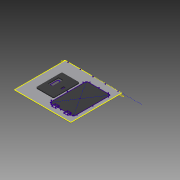
# Autodesk Inventor part: Right_side
Saved by Autodesk Inventor 2015 SP2 (Build 190223200, 223)
## iProperties
Created: 2016-11-11
Part Number: Right_side
Material: Generic
Document SubType Name: Modeling
Designer: Yann Cesbron
Density: 1 g/cm^3
Appearance: Default
Mass: 3388.49 g
Surface Area: 7563.24 cm^2
Volume: 3388.49 cm^3
Material: Perspex Black 9961 -10 mm
Author: Yann Cesbron
Autodesk Inventor part; units mm, degrees
ref_plane "YZ Plane" through (0, 0, 0) normal (1, 0, 0) x (0, 1, 0)
ref_plane "XZ Plane" through (0, 0, 0) normal (0, 1, 0) x (-1, 0, 0)
ref_plane "XY Plane" through (0, 0, 0) normal (0, 0, 1) x (1, 0, 0)
ref_plane "Work Plane1" through (5.6805, -10.8989, 0) normal (0, 0, 1) x (1, 0, 0)
sketch "Sketch1" plane through (5.6805, -10.8989, 0) normal (0, 0, 1) x (1, 0, 0)
  line L0 (-5.6805, 20.8989) -> (604.3195, 20.8989)
  line L1 (604.3195, 20.8989) -> (604.3195, -529.1011)
  line L2 (604.3195, -529.1011) -> (-5.6805, -529.1011)
  line L3 (-5.6805, -529.1011) -> (-5.6805, 20.8989)
  point P0 (-5.6805, 10.8989)
  dimension "d0" = 610
  dimension "d1" = 550
  dimension "d2" = 610
  dimension "d3" = 10
  constraints: 8 end point, 2 parallel, 1 horizontal, 1 perpendicular
  measures "d0" distance of L1.end L2.end
  measures "d1" distance of L0.end L1.end
  measures "d2" distance from line of point (-5.681, 10.899) L1
  measures "d3" distance from line of point (-5.681, 10.899) L0
extrude "Extrusion1" add sketch "Sketch1" along normal blind 10
sketch "Cut_out_right" plane through (5.6805, -10.8989, 10) normal (0, 0, 1) x (1, 0, 0)
  line L0 (604.3195, 20.8989) -> (-5.6805, 20.8989) projected
  line L1 (-5.6805, -529.1011) -> (604.3195, -529.1011) projected
  line L2 (274.3195, 20.8989) -> (824.3195, 20.8989) construction
  line L3 (-5.6805, 20.8989) -> (-5.6805, -529.1011) projected
  line L4 (264.3195, -134.1011) -> (124.3195, -134.1011)
  line L5 (114.3195, -144.1011) -> (114.3195, -374.1011)
  line L6 (124.3195, -384.1011) -> (264.3195, -384.1011)
  line L7 (274.3195, -374.1011) -> (274.3195, -144.1011)
  line L8 (274.3195, -134.1011) -> (114.3195, -384.1011) construction
  line L9 (114.3195, -134.1011) -> (274.3195, -384.1011) construction
  arc A0 (264.3195, -384.1011) -> (274.3195, -374.1011) centre (264.3195, -374.1011) ccw
  arc A1 (274.3195, -144.1011) -> (264.3195, -134.1011) centre (264.3195, -144.1011) ccw
  arc A2 (124.3195, -134.1011) -> (114.3195, -144.1011) centre (124.3195, -144.1011) ccw
  arc A3 (114.3195, -374.1011) -> (124.3195, -384.1011) centre (124.3195, -374.1011) ccw
  line L10 (314.3195, -459.1011) -> (554.3195, -459.1011)
  line L11 (564.3195, -449.1011) -> (564.3195, -69.1011)
  line L12 (554.3195, -59.1011) -> (314.3195, -59.1011)
  line L13 (304.3195, -69.1011) -> (304.3195, -449.1011)
  line L14 (304.3195, -459.1011) -> (564.3195, -59.1011) construction
  line L15 (564.3195, -459.1011) -> (304.3195, -59.1011) construction
  line L16 (604.3195, 20.8989) -> (604.3195, -529.1011) projected
  arc A4 (304.3195, -449.1011) -> (314.3195, -459.1011) centre (314.3195, -449.1011) ccw
  arc A5 (564.3195, -69.1011) -> (554.3195, -59.1011) centre (554.3195, -69.1011) ccw
  arc A6 (314.3195, -59.1011) -> (304.3195, -69.1011) centre (314.3195, -69.1011) ccw
  arc A7 (554.3195, -459.1011) -> (564.3195, -449.1011) centre (554.3195, -449.1011) ccw
  circle A8 centre (281.8195, -149.1011) radius 1.65
  circle A9 centre (259.3195, -126.6011) radius 1.65
  circle A10 centre (281.8195, -369.1011) radius 1.65
  circle A11 centre (281.8195, -259.1011) radius 1.65
  circle A12 centre (194.3195, -126.6011) radius 1.65
  circle A13 centre (129.3195, -126.6011) radius 1.65
  circle A14 centre (106.8195, -149.1011) radius 1.65
  circle A15 centre (106.8195, -259.1011) radius 1.65
  circle A16 centre (106.8195, -369.1011) radius 1.65
  circle A17 centre (129.3195, -391.6011) radius 1.65
  circle A18 centre (259.3195, -391.6011) radius 1.65
  circle A19 centre (194.3195, -391.6011) radius 1.65
  circle A20 centre (352.9195, -471.8011) radius 1.65
  circle A21 centre (384.7195, -471.8011) radius 1.65
  circle A22 centre (515.7195, -471.8011) radius 1.65
  circle A23 centre (483.9195, -471.8011) radius 1.65
  circle A24 centre (534.3195, -466.6011) radius 1.65
  circle A25 centre (434.3195, -466.6011) radius 1.65
  circle A26 centre (334.3195, -466.6011) radius 1.65
  circle A27 centre (296.8195, -429.1011) radius 1.65
  circle A28 centre (296.8195, -259.1011) radius 1.65
  circle A29 centre (296.8195, -89.1011) radius 1.65
  circle A30 centre (334.3195, -51.6011) radius 1.65
  circle A31 centre (434.3195, -51.6011) radius 1.65
  circle A32 centre (534.3195, -51.6011) radius 1.65
  circle A33 centre (571.8195, -89.1011) radius 1.65
  circle A34 centre (571.8195, -259.1011) radius 1.65
  circle A35 centre (571.8195, -429.1011) radius 1.65
  circle A36 centre (569.3195, 15.8989) radius 2.25
  circle A37 centre (434.3195, 15.8989) radius 2.25
  circle A38 centre (299.3195, 15.8989) radius 2.25
  circle A39 centre (164.3195, 15.8989) radius 2.25
  circle A40 centre (29.3195, 15.8989) radius 2.25
  point P0 (-5.6805, 10.8989)
  point P1 (194.3195, -259.1011)
  point P2 (434.3195, -259.1011)
  dimension "d29" = 160
  dimension "d30" = 250
  dimension "d31" = 280
  dimension "d32" = 155
  dimension "d33" = 10
  dimension "d34" = 260
  dimension "d35" = 400
  dimension "d36" = 40
  dimension "d37" = 80
  dimension "d38" = 10
  dimension "d39" = 310
  dimension "d43" = 30
  dimension "d44" = 3.3
  dimension "d45" = 7.5
  dimension "d46" = 15
  dimension "d47" = 3.3
  dimension "d48" = 7.5
  dimension "d49" = 15
  dimension "d64" = 3.3
  dimension "d65" = 3.3
  dimension "d66" = 3.3
  dimension "d67" = 3.3
  dimension "d68" = 3.3
  dimension "d69" = 3.3
  dimension "d70" = 3.3
  dimension "d71" = 3.3
  dimension "d72" = 3.3
  dimension "d73" = 3.3
  dimension "d74" = 7.5
  dimension "d75" = 7.5
  dimension "d76" = 7.5
  dimension "d77" = 7.5
  dimension "d78" = 7.5
  dimension "d79" = 7.5
  dimension "d80" = 7.5
  dimension "d81" = 7.5
  dimension "d82" = 7.5
  dimension "d83" = 7.5
  dimension "d84" = 15
  dimension "d85" = 15
  dimension "d86" = 15
  dimension "d87" = 15
  dimension "d88" = 15
  dimension "d89" = 15
  dimension "d90" = 125
  dimension "d91" = 125
  dimension "d92" = 80
  dimension "d93" = 80
  dimension "d169" = 3.3
  dimension "d170" = 3.3
  dimension "d171" = 3.3
  dimension "d172" = 3.3
  dimension "d173" = 31.8
  dimension "d174" = 31.8
  dimension "d175" = 48.6
  dimension "d176" = 48.6
  dimension "d177" = 12.7
  dimension "d178" = 12.7
  dimension "d179" = 12.7
  dimension "d180" = 12.7
  dimension "d181" = 3.3
  dimension "d182" = 3.3
  dimension "d183" = 3.3
  dimension "d184" = 3.3
  constraints: 41 centre point, 26 end point, 17 point on line, 16 point on circle, 16 tangent, 6 equal radius, 4 midpoint, 4 parallel, 3 horizontal, 2 perpendicular
  measures "d29" distance of L9.end L8.end
  measures "d30" distance of L8.end L9.start
  measures "d31" distance between parallel lines of L3 L7
  measures "d32" distance between parallel lines of L0 L4
  measures "d33" radius of A0
  measures "d34" distance of L15.end L14.end
  measures "d35" distance of L14.end L15.start
  measures "d36" distance between parallel lines of L16 L11
  measures "d37" distance between parallel lines of L0 L12
  measures "d38" radius of A4
  measures "d39" distance between parallel lines of L3 L13
  measures "d43" distance between parallel lines of L7 L13
  measures "d44" diameter of A8
  measures "d45" distance from line of L7 A8.centre
  measures "d46" distance from line of A8.centre L4
  measures "d47" diameter of A9
  measures "d48" distance from line of L4 A9.centre
  measures "d49" distance from line of A9.centre L7
  measures "d64" diameter of A10
  measures "d65" diameter of A11
  measures "d66" diameter of A12
  measures "d67" diameter of A13
  measures "d68" diameter of A14
  measures "d69" diameter of A15
  measures "d70" diameter of A16
  measures "d71" diameter of A17
  measures "d72" diameter of A18
  measures "d73" diameter of A19
  measures "d74" distance from line of L4 A12.centre
  measures "d75" distance from line of L4 A13.centre
  measures "d76" distance from line of L7 A11.centre
  measures "d77" distance from line of L5 A14.centre
  measures "d78" distance from line of L5 A15.centre
  measures "d79" distance from line of L5 A16.centre
  measures "d80" distance from line of L6 A17.centre
  measures "d81" distance from line of L6 A19.centre
  measures "d82" distance from line of L7 A10.centre
  measures "d83" distance from line of L6 A18.centre
  measures "d84" distance from line of L7 A18.centre
  measures "d85" distance from line of L5 A17.centre
  measures "d86" distance from line of L5 A13.centre
  measures "d87" distance from line of L4 A14.centre
  measures "d88" distance from line of L6 A16.centre
  measures "d89" distance from line of L6 A10.centre
  measures "d90" distance from line of L4 A11.centre
  measures "d91" distance from line of L6 A15.centre
  measures "d92" distance from line of L5 A12.centre
  measures "d93" distance from line of L7 A19.centre
  measures "d169" diameter of A20
  measures "d170" diameter of A21
  measures "d171" diameter of A22
  measures "d172" diameter of A23
  measures "d173" distance of A23.centre A22.centre
  measures "d174" distance of A20.centre A21.centre
  measures "d175" distance from line of A20.centre L13
  measures "d176" distance from line of A22.centre L11
  measures "d177" distance from line of L10 A22.centre
  measures "d178" distance from line of L10 A23.centre
  measures "d179" distance from line of L10 A21.centre
  measures "d180" distance from line of L10 A20.centre
  measures "d181" diameter of A24
  measures "d182" diameter of A25
  measures "d183" diameter of A26
  measures "d184" diameter of A27
sketch "Panel_right_holes_right" plane through (0, -540, 0) normal (0, -1, 0) x (1, 0, 0)
  circle A0 centre (575, 5) radius 1.65
  circle A1 centre (440, 5) radius 1.65
  circle A2 centre (305, 5) radius 1.65
  circle A3 centre (170, 5) radius 1.65
  circle A4 centre (35, 5) radius 1.65
  line L0 (0, 0) -> (0, 10) projected
  line L1 (610, 0) -> (0, 0) projected
  line L2 (610, 0) -> (610, 10) projected
  dimension "d256" = 3.3
  dimension "d257" = 3.3
  dimension "d258" = 3.3
  dimension "d259" = 3.3
  dimension "d260" = 3.3
  dimension "d261" = 35
  dimension "d262" = 5
  dimension "d263" = 5
  dimension "d264" = 135
  dimension "d265" = 135
  dimension "d266" = 5
  dimension "d268" = 5
  dimension "d269" = 35
  dimension "d270" = 5
  dimension "d271" = 135
  constraints: 5 centre point
  measures "d256" diameter of A0
  measures "d257" diameter of A1
  measures "d258" diameter of A2
  measures "d259" diameter of A3
  measures "d260" diameter of A4
  measures "d261" distance from line of L0 A4.centre
  measures "d262" distance from line of L1 A4.centre
  measures "d263" distance from line of L1 A3.centre
  measures "d264" distance of A4.centre A3.centre
  measures "d265" distance of A2.centre A3.centre
  measures "d266" distance from line of L1 A2.centre
  measures "d268" distance from line of L1 A1.centre
  measures "d269" distance from line of L2 A0.centre
  measures "d270" distance from line of L1 A0.centre
  measures "d271" distance of A1.centre A0.centre
sketch "Panel_top_holes_right" plane through (610, -540, 0) normal (1, 0, 0) x (0, 0, -1)
  circle A0 centre (-5, 515) radius 1.65
  circle A1 centre (-5, 355) radius 1.65
  circle A2 centre (-5, 195) radius 1.65
  circle A3 centre (-5, 35) radius 1.65
  line L0 (-10, 0) -> (-10, 550) projected
  line L1 (0, 0) -> (-10, 0) projected
  line L2 (0, 550) -> (-10, 550) projected
  point P0 (0, 540)
  dimension "d272" = 3.3
  dimension "d273" = 3.3
  dimension "d274" = 3.3
  dimension "d275" = 3.3
  dimension "d276" = 5
  dimension "d277" = 35
  dimension "d278" = 5
  dimension "d279" = 160
  dimension "d280" = 5
  dimension "d281" = 5
  dimension "d282" = 35
  dimension "d283" = 160
  dimension "d284" = 160
  constraints: 4 centre point
  measures "d272" diameter of A0
  measures "d273" diameter of A1
  measures "d274" diameter of A2
  measures "d275" diameter of A3
  measures "d276" distance from line of L0 A3.centre
  measures "d277" distance from line of L1 A3.centre
  measures "d278" distance from line of L0 A2.centre
  measures "d279" distance of A3.centre A2.centre
  measures "d280" distance from line of L0 A0.centre
  measures "d281" distance from line of L0 A1.centre
  measures "d282" distance from line of A0.centre L2
  measures "d283" distance of A1.centre A0.centre
  measures "d284" distance of A2.centre A1.centre
extrude "Extrusion2" cut sketch "Cut_out_right" against normal blind 10 keep common part
extrude "Extrusion6" cut sketch "Panel_top_holes_right" against normal blind 15
extrude "Extrusion5" cut sketch "Panel_right_holes_right" against normal blind 15
sketch "Bracket_holes_right" plane through (5.6805, -10.8989, 10) normal (0, 0, 1) x (1, 0, 0)
  line L0 (-5.6805, 20.8989) -> (-5.6805, -529.1011) projected
  line L1 (-5.6805, -529.1011) -> (604.3195, -529.1011) projected
  line L2 (604.3195, 20.8989) -> (-5.6805, 20.8989) projected
  point P0 (-5.6805, 10.8989)
  point P1 (1.8195, -109.1011)
  point P2 (1.8195, -409.1011)
  dimension "d562" = 7.5
  dimension "d563" = 120
  dimension "d564" = 7.5
  dimension "d565" = 130
  measures "d562" distance from line of L0 point (1.819, -409.101)
  measures "d563" distance from line of L1 point (1.819, -409.101)
  measures "d564" distance from line of L0 point (1.819, -109.101)
  measures "d565" distance from line of L2 point (1.819, -109.101)
hole "Bracket_holes_right_1" at (7.5, -120, 10) at (7.5, -420, 10) direction (0, 0, -1) diameter 3.3 end through all
sketch "CRISP+X-motor" plane through (5.6805, -10.8989, 10) normal (0, 0, 1) x (1, 0, 0)
  circle A0 centre (250.3195, -259.1011) radius 8
  line L0 (138.3195, -204.1011) -> (168.4695, -204.1011)
  line L1 (168.4695, -204.1011) -> (168.4695, -289.2011)
  line L2 (168.4695, -289.2011) -> (138.3195, -289.2011)
  line L3 (138.3195, -289.2011) -> (138.3195, -204.1011)
  line L4 (604.3195, 20.8989) -> (-5.6805, 20.8989) projected
  line L5 (-5.6805, 20.8989) -> (-5.6805, -529.1011) projected
  line L6 (242.7195, -242.6011) -> (257.9195, -242.6011)
  line L7 (257.9195, -242.6011) -> (257.9195, -275.6011)
  line L8 (257.9195, -275.6011) -> (242.7195, -275.6011)
  line L9 (242.7195, -275.6011) -> (242.7195, -242.6011)
  line L10 (242.7195, -242.6011) -> (257.9195, -275.6011) construction
  line L11 (257.9195, -242.6011) -> (242.7195, -275.6011) construction
  point P0 (-5.6805, 10.8989)
  dimension "d19" = 16
  dimension "d20" = 30.15
  dimension "d21" = 85.1
  dimension "d22" = 280
  dimension "d23" = 256
  dimension "d24" = 225
  dimension "d25" = 144
  dimension "d41" = 33
  dimension "d42" = 15.2
  constraints: 20 end point, 4 parallel, 2 horizontal, 2 midpoint, 2 perpendicular, 1 centre point
  measures "d19" diameter of A0
  measures "d20" distance of L1.end L2.end
  measures "d21" distance of L0.end L1.end
  measures "d22" distance from line of L4 A0.centre
  measures "d23" distance from line of L5 A0.centre
  measures "d24" distance from line of L4 L0.start
  measures "d25" distance between parallel lines of L5 L3
  measures "d41" distance of L6.end L7.end
  measures "d42" distance between parallel lines of L9 L7
sketch "Hinges_right" plane through (5.6805, -10.8989, 10) normal (0, 0, 1) x (1, 0, 0)
  line L0 (524.3195, -481.1011) -> (475.3195, -481.1011)
  line L1 (475.3195, -481.1011) -> (475.3195, -437.1011)
  line L2 (475.3195, -437.1011) -> (524.3195, -437.1011)
  line L3 (524.3195, -437.1011) -> (524.3195, -481.1011)
  line L4 (344.3195, -481.1011) -> (393.3195, -481.1011)
  line L5 (393.3195, -481.1011) -> (393.3195, -437.1011)
  line L6 (393.3195, -437.1011) -> (344.3195, -437.1011)
  line L7 (344.3195, -437.1011) -> (344.3195, -481.1011)
  line L8 (-5.6805, -529.1011) -> (604.3195, -529.1011) projected
  line L9 (604.3195, -529.1011) -> (604.3195, 20.8989) projected
  circle A0 centre (515.7195, -446.4011) radius 2.25
  circle A1 centre (483.9195, -446.4011) radius 2.25
  circle A2 centre (515.7195, -471.8011) radius 2.25
  circle A3 centre (483.9195, -471.8011) radius 2.25
  circle A4 centre (352.9195, -471.8011) radius 2.25
  circle A5 centre (352.9195, -446.4011) radius 2.25
  circle A6 centre (384.7195, -446.4011) radius 2.25
  circle A7 centre (384.7195, -471.8011) radius 2.25
  point P0 (-5.6805, 10.8989)
  dimension "d130" = 49
  dimension "d131" = 44
  dimension "d132" = 49
  dimension "d133" = 44
  dimension "d143" = 80
  dimension "d144" = 260
  dimension "d145" = 4.5
  dimension "d146" = 4.5
  dimension "d147" = 4.5
  dimension "d148" = 4.5
  dimension "d149" = 4.5
  dimension "d150" = 4.5
  dimension "d151" = 4.5
  dimension "d152" = 4.5
  dimension "d153" = 9.3
  dimension "d154" = 9.3
  dimension "d155" = 8.6
  dimension "d156" = 8.6
  dimension "d157" = 8.6
  dimension "d158" = 8.6
  dimension "d159" = 9.3
  dimension "d160" = 9.3
  dimension "d161" = 8.6
  dimension "d162" = 8.6
  dimension "d163" = 8.6
  dimension "d164" = 8.6
  dimension "d165" = 9.3
  dimension "d166" = 9.3
  dimension "d167" = 9.3
  dimension "d168" = 9.3
  dimension "d239" = 48
  dimension "d240" = 48
  constraints: 16 end point, 8 centre point, 4 parallel, 2 horizontal, 2 perpendicular
  measures "d130" distance of L1.end L2.end
  measures "d131" distance of L0.end L1.end
  measures "d132" distance of L6.end L5.end
  measures "d133" distance of L5.end L4.end
  measures "d143" distance between parallel lines of L9 L3
  measures "d144" distance between parallel lines of L7 L9
  measures "d145" diameter of A0
  measures "d146" diameter of A1
  measures "d147" diameter of A2
  measures "d148" diameter of A3
  measures "d149" diameter of A4
  measures "d150" diameter of A5
  measures "d151" diameter of A6
  measures "d152" diameter of A7
  measures "d153" distance from line of L0 A2.centre
  measures "d154" distance from line of L0 A3.centre
  measures "d155" distance from line of L3 A2.centre
  measures "d156" distance from line of L3 A0.centre
  measures "d157" distance from line of L1 A1.centre
  measures "d158" distance from line of L1 A3.centre
  measures "d159" distance from line of L2 A0.centre
  measures "d160" distance from line of L2 A1.centre
  measures "d161" distance from line of L5 A6.centre
  measures "d162" distance from line of L5 A7.centre
  measures "d163" distance from line of L7 A5.centre
  measures "d164" distance from line of L7 A4.centre
  measures "d165" distance from line of L4 A4.centre
  measures "d166" distance from line of L6 A5.centre
  measures "d167" distance from line of L6 A6.centre
  measures "d168" distance from line of L4 A7.centre
  measures "d239" distance between parallel lines of L8 L0
  measures "d240" distance between parallel lines of L8 L4
sketch "Flange_right" plane through (5.6805, -10.8989, 10) normal (0, 0, 1) x (1, 0, 0)
  line L0 (279.3195, -119.1011) -> (109.3195, -119.1011)
  line L1 (99.3195, -129.1011) -> (99.3195, -389.1011)
  line L2 (109.3195, -399.1011) -> (279.3195, -399.1011)
  line L3 (289.3195, -389.1011) -> (289.3195, -129.1011)
  line L4 (289.3195, -119.1011) -> (99.3195, -399.1011) construction
  line L5 (99.3195, -119.1011) -> (289.3195, -399.1011) construction
  line L6 (604.3195, 20.8989) -> (-5.6805, 20.8989) projected
  line L7 (-5.6805, 20.8989) -> (-5.6805, -529.1011) projected
  line L8 (128.3195, -184.1011) -> (178.4695, -184.1011)
  line L9 (178.4695, -184.1011) -> (178.4695, -299.2011)
  line L10 (178.4695, -299.2011) -> (128.3195, -299.2011)
  line L11 (128.3195, -299.2011) -> (128.3195, -184.1011)
  line L12 (260.3195, -240.1011) -> (240.3195, -240.1011)
  line L13 (240.3195, -240.1011) -> (240.3195, -278.1011)
  line L14 (240.3195, -278.1011) -> (260.3195, -278.1011)
  line L15 (260.3195, -278.1011) -> (260.3195, -240.1011)
  line L16 (260.3195, -240.1011) -> (240.3195, -278.1011) construction
  line L17 (240.3195, -240.1011) -> (260.3195, -278.1011) construction
  circle A0 centre (194.3195, -126.6011) radius 2.25
  circle A1 centre (259.3195, -126.6011) radius 2.25
  circle A2 centre (281.8195, -149.1011) radius 2.25
  circle A3 centre (281.8195, -259.1011) radius 2.25
  circle A4 centre (281.8195, -369.1011) radius 2.25
  circle A5 centre (259.3195, -391.6011) radius 2.25
  circle A6 centre (194.3195, -391.6011) radius 2.25
  circle A7 centre (129.3195, -391.6011) radius 2.25
  circle A8 centre (106.8195, -369.1011) radius 2.25
  circle A9 centre (106.8195, -259.1011) radius 2.25
  circle A10 centre (106.8195, -149.1011) radius 2.25
  circle A11 centre (129.3195, -126.6011) radius 2.25
  arc A12 (289.3195, -129.1011) -> (279.3195, -119.1011) centre (279.3195, -129.1011) ccw
  arc A13 (279.3195, -399.1011) -> (289.3195, -389.1011) centre (279.3195, -389.1011) ccw
  arc A14 (109.3195, -119.1011) -> (99.3195, -129.1011) centre (109.3195, -129.1011) ccw
  arc A15 (99.3195, -389.1011) -> (109.3195, -399.1011) centre (109.3195, -389.1011) ccw
  point P0 (-5.6805, 10.8989)
  point P1 (194.3195, -259.1011)
  point P2 (250.3195, -259.1011)
  dimension "d51" = 190
  dimension "d52" = 280
  dimension "d53" = 280
  dimension "d54" = 200
  dimension "d55" = 50.15
  dimension "d56" = 65
  dimension "d57" = 29
  dimension "d58" = 115.1
  dimension "d59" = 20
  dimension "d60" = 38
  dimension "d62" = 39
  dimension "d63" = 140
  dimension "d94" = 4.5
  dimension "d95" = 4.5
  dimension "d96" = 4.5
  dimension "d97" = 4.5
  dimension "d98" = 4.5
  dimension "d99" = 4.5
  dimension "d100" = 4.5
  dimension "d101" = 4.5
  dimension "d102" = 4.5
  dimension "d103" = 4.5
  dimension "d104" = 4.5
  dimension "d105" = 4.5
  dimension "d106" = 7.5
  dimension "d107" = 30
  dimension "d108" = 7.5
  dimension "d109" = 140
  dimension "d110" = 7.5
  dimension "d111" = 30
  dimension "d112" = 7.5
  dimension "d113" = 7.5
  dimension "d114" = 7.5
  dimension "d115" = 7.5
  dimension "d116" = 7.5
  dimension "d117" = 30
  dimension "d118" = 30
  dimension "d119" = 30
  dimension "d120" = 30
  dimension "d121" = 7.5
  dimension "d122" = 7.5
  dimension "d123" = 7.5
  dimension "d124" = 7.5
  dimension "d125" = 30
  dimension "d126" = 30
  dimension "d127" = 140
  dimension "d128" = 95
  dimension "d129" = 95
  dimension "d217" = 10
  constraints: 32 end point, 16 centre point, 8 point on circle, 8 point on line, 8 tangent, 6 parallel, 4 midpoint, 3 equal radius, 3 horizontal, 3 perpendicular
  measures "d51" distance of L5.end L4.end
  measures "d52" distance of L4.end L5.start
  measures "d53" distance from line of L6 point (194.319, -259.101)
  measures "d54" distance from line of L7 point (194.319, -259.101)
  measures "d55" distance of L9.end L10.end
  measures "d56" distance between parallel lines of L0 L8
  measures "d57" distance between parallel lines of L1 L11
  measures "d58" distance between parallel lines of L10 L8
  measures "d59" distance of L14.end L13.end
  measures "d60" distance of L13.end L12.end
  measures "d62" distance from line of L3 point (250.319, -259.101)
  measures "d63" distance from line of L0 point (250.319, -259.101)
  measures "d94" diameter of A0
  measures "d95" diameter of A1
  measures "d96" diameter of A2
  measures "d97" diameter of A3
  measures "d98" diameter of A4
  measures "d99" diameter of A5
  measures "d100" diameter of A6
  measures "d101" diameter of A7
  measures "d102" diameter of A8
  measures "d103" diameter of A9
  measures "d104" diameter of A10
  measures "d105" diameter of A11
  measures "d106" distance from line of L3 A2.centre
  measures "d107" distance from line of L0 A2.centre
  measures "d108" distance from line of L3 A3.centre
  measures "d109" distance from line of L0 A3.centre
  measures "d110" distance from line of L3 A4.centre
  measures "d111" distance from line of L2 A4.centre
  measures "d112" distance from line of L2 A5.centre
  measures "d113" distance from line of L2 A6.centre
  measures "d114" distance from line of L0 A1.centre
  measures "d115" distance from line of L0 A0.centre
  measures "d116" distance from line of L0 A11.centre
  measures "d117" distance from line of L3 A1.centre
  measures "d118" distance from line of L1 A11.centre
  measures "d119" distance from line of L3 A5.centre
  measures "d120" distance from line of L1 A7.centre
  measures "d121" distance from line of L2 A7.centre
  measures "d122" distance from line of L1 A8.centre
  measures "d123" distance from line of L1 A10.centre
  measures "d124" distance from line of L1 A9.centre
  measures "d125" distance from line of A10.centre L0
  measures "d126" distance from line of L2 A8.centre
  measures "d127" distance from line of L2 A9.centre
  measures "d128" distance from line of L3 A6.centre
  measures "d129" distance from line of L1 A0.centre
  measures "d217" radius of A12
sketch "Door_right" plane through (5.6805, -10.8989, 10) normal (0, 0, 1) x (1, 0, 0)
  line L0 (554.3195, -457.1011) -> (314.3195, -457.1011)
  line L1 (306.3195, -449.1011) -> (306.3195, -69.1011)
  line L2 (314.3195, -61.1011) -> (554.3195, -61.1011)
  line L3 (562.3195, -69.1011) -> (562.3195, -449.1011)
  line L4 (562.3195, -457.1011) -> (306.3195, -61.1011) construction
  line L5 (306.3195, -457.1011) -> (562.3195, -61.1011) construction
  arc A0 (562.3195, -69.1011) -> (554.3195, -61.1011) centre (554.3195, -69.1011) ccw
  arc A1 (314.3195, -61.1011) -> (306.3195, -69.1011) centre (314.3195, -69.1011) ccw
  arc A2 (306.3195, -449.1011) -> (314.3195, -457.1011) centre (314.3195, -449.1011) ccw
  arc A3 (554.3195, -457.1011) -> (562.3195, -449.1011) centre (554.3195, -449.1011) ccw
  circle A4 centre (515.7195, -446.4011) radius 1.65
  circle A5 centre (483.9195, -446.4011) radius 1.65
  circle A6 centre (384.7195, -446.4011) radius 1.65
  circle A7 centre (352.9195, -446.4011) radius 1.65
  line L6 (-5.6805, 20.8989) -> (-5.6805, -529.1011) projected
  line L7 (604.3195, 20.8989) -> (-5.6805, 20.8989) projected
  point P0 (-5.6805, 10.8989)
  point P1 (434.3195, -259.1011)
  dimension "d218" = 256
  dimension "d219" = 396
  dimension "d220" = 8
  dimension "d221" = 8
  dimension "d222" = 8
  dimension "d223" = 8
  dimension "d224" = 3.3
  dimension "d225" = 3.3
  dimension "d226" = 3.3
  dimension "d227" = 3.3
  dimension "d228" = 10.7
  dimension "d229" = 10.7
  dimension "d230" = 31.8
  dimension "d231" = 10.7
  dimension "d232" = 10.7
  dimension "d233" = 31.8
  dimension "d234" = 46.6
  dimension "d235" = 46.6
  dimension "d236" = 440
  dimension "d237" = 280
  constraints: 12 end point, 8 centre point, 8 point on circle, 8 point on line, 8 tangent, 2 midpoint, 2 parallel, 1 horizontal, 1 perpendicular
  measures "d218" distance of L4.end L5.end
  measures "d219" distance of L5.start L4.end
  measures "d220" radius of A0
  measures "d221" radius of A1
  measures "d222" radius of A2
  measures "d223" radius of A3
  measures "d224" diameter of A4
  measures "d225" diameter of A5
  measures "d226" diameter of A6
  measures "d227" diameter of A7
  measures "d228" distance from line of L0 A4.centre
  measures "d229" distance from line of L0 A5.centre
  measures "d230" distance of A4.centre A5.centre
  measures "d231" distance from line of L0 A6.centre
  measures "d232" distance from line of L0 A7.centre
  measures "d233" distance of A7.centre A6.centre
  measures "d234" distance from line of L1 A7.centre
  measures "d235" distance from line of L3 A4.centre
  measures "d236" distance from line of L6 point (434.319, -259.101)
  measures "d237" distance from line of L7 point (434.319, -259.101)
extrude "Extrusion3" add sketch "Door_right" against normal blind 10 separate body
extrude "Extrusion4" add sketch "Flange_right" along normal blind 10 separate body
sketch "Door_hole_right" plane through (5.6805, -10.8989, 0) normal (0, 0, -1) x (-1, 0, 0)
  line L0 (-306.3195, -449.1011) -> (-306.3195, -69.1011) projected
  line L1 (-314.3195, -61.1011) -> (-554.3195, -61.1011) projected
  point P0 (5.6805, 10.8989)
  point P1 (-434.3195, -74.1011)
  dimension "d333" = 128
  dimension "d334" = 13
  measures "d333" distance from line of L0 point (-434.319, -74.101)
  measures "d334" distance from line of L1 point (-434.319, -74.101)
hole "CSK_Door_hole_right" at (440, -85, 0) direction (0, 0, 1) diameter 7 end through all countersink diameter 12.6 countersink angle 90 bodies 2 clearance for "Countersunk Flat Head Screw DIN EN ISO 2009" size "M6" standard "DIN"
sketch "Door_flanges_right" plane through (5.6805, -10.8989, 0) normal (0, 0, -1) x (-1, 0, 0)
  line L0 (-289.3195, -70.1011) -> (-314.3195, -70.1011)
  line L1 (-314.3195, -70.1011) -> (-314.3195, -448.1011)
  line L2 (-314.3195, -448.1011) -> (-289.3195, -448.1011)
  line L3 (-289.3195, -448.1011) -> (-289.3195, -70.1011)
  line L4 (-304.3195, -449.1011) -> (-304.3195, -69.1011) projected
  line L5 (-579.3195, -449.1011) -> (-289.3195, -449.1011)
  line L6 (-289.3195, -449.1011) -> (-289.3195, -474.1011)
  line L7 (-289.3195, -474.1011) -> (-579.3195, -474.1011)
  line L8 (-579.3195, -474.1011) -> (-579.3195, -449.1011)
  line L9 (-554.3195, -459.1011) -> (-314.3195, -459.1011) projected
  line L10 (-579.3195, -44.1011) -> (-289.3195, -44.1011)
  line L11 (-289.3195, -44.1011) -> (-289.3195, -69.1011)
  line L12 (-579.3195, -69.1011) -> (-579.3195, -44.1011)
  line L13 (-314.3195, -59.1011) -> (-554.3195, -59.1011) projected
  line L14 (-579.3195, -70.1011) -> (-554.3195, -70.1011)
  line L15 (-554.3195, -70.1011) -> (-554.3195, -448.1011)
  line L16 (-554.3195, -448.1011) -> (-579.3195, -448.1011)
  line L17 (-579.3195, -448.1011) -> (-579.3195, -70.1011)
  line L18 (-564.3195, -69.1011) -> (-564.3195, -449.1011) projected
  circle A0 centre (-571.8195, -89.1011) radius 2.25
  circle A1 centre (-571.8195, -259.1011) radius 2.25
  circle A2 centre (-571.8195, -429.1011) radius 2.25
  circle A3 centre (-534.3195, -466.6011) radius 2.25
  circle A4 centre (-434.3195, -466.6011) radius 2.25
  circle A5 centre (-334.3195, -466.6011) radius 1.65 projected
  circle A6 centre (-296.8195, -429.1011) radius 2.25
  circle A7 centre (-296.8195, -259.1011) radius 2.25
  circle A8 centre (-296.8195, -89.1011) radius 2.25
  circle A9 centre (-334.3195, -51.6011) radius 2.25
  circle A10 centre (-434.3195, -51.6011) radius 2.25
  circle A11 centre (-534.3195, -51.6011) radius 2.25
  circle A12 centre (-334.3195, -466.6011) radius 2.25
  line L19 (-424.3195, -69.1011) -> (-424.3195, -61.1011)
  line L20 (-424.3195, -61.1011) -> (-444.3195, -61.1011)
  line L21 (-444.3195, -61.1011) -> (-444.3195, -69.1011)
  line L22 (-289.3195, -69.1011) -> (-424.3195, -69.1011)
  line L23 (-444.3195, -69.1011) -> (-579.3195, -69.1011)
  circle A13 centre (-451.8195, -61.6011) radius 1.65
  circle A14 centre (-416.8195, -61.6011) radius 1.65
  point P0 (5.6805, 10.8989)
  dimension "d295" = 25
  dimension "d297" = 15
  dimension "d298" = 290
  dimension "d299" = 25
  dimension "d301" = 290
  dimension "d302" = 25
  dimension "d304" = 15
  dimension "d305" = 15
  dimension "d306" = 25
  dimension "d308" = 15
  dimension "d342" = 15
  dimension "d343" = 15
  dimension "d344" = 1
  dimension "d345" = 1
  dimension "d348" = 378
  dimension "d349" = 378
  dimension "d350" = 4.5
  dimension "d351" = 4.5
  dimension "d352" = 4.5
  dimension "d353" = 4.5
  dimension "d354" = 4.5
  dimension "d356" = 4.5
  dimension "d357" = 4.5
  dimension "d358" = 4.5
  dimension "d359" = 4.5
  dimension "d360" = 4.5
  dimension "d361" = 4.5
  dimension "d362" = 7.5
  dimension "d363" = 7.5
  dimension "d364" = 7.5
  dimension "d365" = 7.5
  dimension "d366" = 7.5
  dimension "d367" = 7.5
  dimension "d368" = 7.5
  dimension "d369" = 7.5
  dimension "d370" = 7.5
  dimension "d372" = 7.5
  dimension "d373" = 7.5
  dimension "d374" = 19
  dimension "d375" = 19
  dimension "d376" = 170
  dimension "d377" = 170
  dimension "d378" = 45
  dimension "d379" = 4.5
  dimension "d380" = 7.5
  dimension "d381" = 45
  dimension "d382" = 100
  dimension "d383" = 19
  dimension "d384" = 170
  dimension "d385" = 19
  dimension "d386" = 45
  dimension "d387" = 100
  dimension "d388" = 45
  dimension "d393" = 20
  dimension "d394" = 8
  dimension "d405" = 135
  dimension "d406" = 135
  dimension "d407" = 25
  dimension "d429" = 3.3
  dimension "d430" = 3.3
  dimension "d431" = 7.5
  dimension "d432" = 7.5
  dimension "d433" = 7.5
  dimension "d434" = 7.5
  constraints: 40 end point, 14 centre point, 10 parallel, 4 horizontal, 4 perpendicular
  measures "d295" distance of L2.end L1.end
  measures "d297" distance between parallel lines of L4 L3
  measures "d298" distance of L6.end L7.end
  measures "d299" distance of L5.end L6.end
  measures "d301" distance of L11.end L12.start
  measures "d302" distance of L10.end L11.end
  measures "d304" distance between parallel lines of L13 L10
  measures "d305" distance between parallel lines of L9 L7
  measures "d306" distance of L15.end L16.end
  measures "d308" distance between parallel lines of L18 L17
  measures "d342" distance from line of L18 L5.start
  measures "d343" distance between parallel lines of L18 L12
  measures "d344" distance between parallel lines of L5 L16
  measures "d345" distance from line of L5 L2.end
  measures "d348" distance between parallel lines of L14 L16
  measures "d349" distance between parallel lines of L0 L2
  measures "d350" diameter of A0
  measures "d351" diameter of A1
  measures "d352" diameter of A2
  measures "d353" diameter of A3
  measures "d354" diameter of A4
  measures "d356" diameter of A6
  measures "d357" diameter of A7
  measures "d358" diameter of A8
  measures "d359" diameter of A9
  measures "d360" diameter of A10
  measures "d361" diameter of A11
  measures "d362" distance from line of L17 A2.centre
  measures "d363" distance from line of L17 A1.centre
  measures "d364" distance from line of L17 A0.centre
  measures "d365" distance from line of L10 A11.centre
  measures "d366" distance from line of L10 A10.centre
  measures "d367" distance from line of L10 A9.centre
  measures "d368" distance from line of L3 A8.centre
  measures "d369" distance from line of L3 A7.centre
  measures "d370" distance from line of L3 A6.centre
  measures "d372" distance from line of L7 A4.centre
  measures "d373" distance from line of L7 A3.centre
  measures "d374" distance from line of L16 A2.centre
  measures "d375" distance from line of L14 A0.centre
  measures "d376" distance of A0.centre A1.centre
  measures "d377" distance of A2.centre A1.centre
  measures "d378" distance from line of L8 A3.centre
  measures "d379" diameter of A12
  measures "d380" distance from line of L7 A12.centre
  measures "d381" distance from line of L6 A12.centre
  measures "d382" distance of A4.centre A5.centre
  measures "d383" distance from line of L2 A6.centre
  measures "d384" distance of A6.centre A7.centre
  measures "d385" distance from line of L0 A8.centre
  measures "d386" distance from line of L11 A9.centre
  measures "d387" distance of A10.centre A9.centre
  measures "d388" distance from line of L12 A11.centre
  measures "d393" distance of L20.end L19.end
  measures "d394" distance of L19.end L19.start
  measures "d405" distance between parallel lines of L21 L12
  measures "d406" distance between parallel lines of L19 L11
  measures "d407" distance between parallel lines of L10 L23
  measures "d429" diameter of A13
  measures "d430" diameter of A14
  measures "d431" distance from line of L23 A13.centre
  measures "d432" distance from line of L22 A14.centre
  measures "d433" distance from line of L19 A14.centre
  measures "d434" distance from line of L21 A13.centre
extrude "Door_flanges_right_1" add sketch "Door_flanges_right" along normal blind 10 separate body contours L5 L6 L7 L8
extrude "Door_flanges_right_2" add sketch "Door_flanges_right" along normal blind 10 separate body contours L18 L14 L15 L16 | L16 L17 L14 L18
extrude "Door_flanges_right_3" add sketch "Door_flanges_right" along normal blind 10 separate body contours L3 L2 L4 L0 | L4 L2 L1 L0
extrude "Door_flanges_right_4" add sketch "Door_flanges_right" along normal blind 10 separate body contours L22 L19 L20 L21 L23 L12 L10 L11
sketch "Magnet_flange_right" plane through (5.6805, -10.8989, -10) normal (0, 0, -1) x (-1, 0, 0)
  line L0 (-444.3195, -84.1011) -> (-424.3195, -84.1011)
  line L1 (-409.3195, -69.1011) -> (-409.3195, -54.1011)
  line L2 (-459.3195, -54.1011) -> (-459.3195, -69.1011)
  line L3 (-444.3195, -84.1011) -> (-444.3195, -69.1011)
  line L4 (-444.3195, -69.1011) -> (-459.3195, -69.1011)
  line L5 (-424.3195, -84.1011) -> (-424.3195, -69.1011)
  line L6 (-424.3195, -69.1011) -> (-409.3195, -69.1011)
  circle A0 centre (-451.8195, -61.6011) radius 2.25
  circle A1 centre (-416.8195, -61.6011) radius 2.25
  arc A2 (-440.3195, -54.1011) -> (-428.3195, -54.1011) centre (-434.3195, -54.1011) ccw
  line L7 (-409.3195, -54.1011) -> (-428.3195, -54.1011)
  line L8 (-440.3195, -54.1011) -> (-459.3195, -54.1011)
  circle A3 centre (-434.3195, -74.1011) radius 1.65
  point P0 (5.6805, 10.8989)
  dimension "d506" = 50
  dimension "d507" = 15
  dimension "d508" = 15
  dimension "d509" = 15
  dimension "d510" = 4.5
  dimension "d511" = 4.5
  dimension "d512" = 7.5
  dimension "d513" = 7.5
  dimension "d516" = 12
  dimension "d517" = 15
  dimension "d518" = 15
  dimension "d519" = 7.5
  dimension "d520" = 7.5
  dimension "d521" = 19
  dimension "d523" = 3.3
  dimension "d524" = 10
  dimension "d525" = 10
  constraints: 18 end point, 4 centre point, 3 parallel, 3 perpendicular, 2 line through centre, 2 point on circle, 1 coincident, 1 horizontal
  measures "d506" distance between parallel lines of L1 L2
  measures "d507" distance between parallel lines of L2 L3
  measures "d508" distance between parallel lines of L1 L5
  measures "d509" distance between parallel lines of L0 L4
  measures "d510" diameter of A0
  measures "d511" diameter of A1
  measures "d512" distance from line of L2 A0.centre
  measures "d513" distance from line of L1 A1.centre
  measures "d516" diameter of A2
  measures "d517" distance between parallel lines of L8 L4
  measures "d518" distance between parallel lines of L7 L6
  measures "d519" distance from line of L4 A0.centre
  measures "d520" distance from line of L6 A1.centre
  measures "d521" distance of L8.start L8.end
  measures "d523" diameter of A3
  measures "d524" distance from line of L3 A3.centre
  measures "d525" distance from line of L0 A3.centre
extrude "Magnet_flange_right_1" add sketch "Magnet_flange_right" along normal blind 10 separate body
